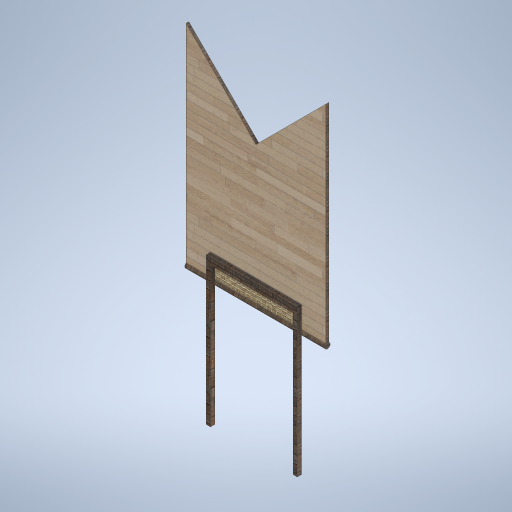
# Autodesk Inventor part: flag
Saved by Autodesk Inventor 2024.2 (Build 282272000, 272)
## iProperties
Created: 2024-05-27
Part Number: flag
Material: 一般
Document SubType Name: Modeling
Designer: user
Density: 1 g/cm^3
Appearance: 預設
Author: user
Autodesk Inventor part; units mm, degrees
ref_plane "YZ Plane" through (0, 0, 0) normal (1, 0, 0) x (0, 1, 0)
ref_plane "XZ Plane" through (0, 0, 0) normal (0, 1, 0) x (-1, 0, 0)
ref_plane "XY Plane" through (0, 0, 0) normal (0, 0, 1) x (1, 0, 0)
sketch "草圖1" plane through (0, 0, 0) normal (0, 0, 1) x (1, 0, 0)
  line L0 (-500, -500) -> (0, -1000)
  line L1 (0, -1000) -> (500, -500)
  line L2 (-500, -500) -> (-500, -2000)
  line L3 (-500, -2000) -> (500, -2000)
  line L4 (500, -2000) -> (500, -500)
  point P0 (0, 0)
  dimension "d2" = 1500
  dimension "d3" = 1000
  constraints: 10 end point, 2 perpendicular, 1 vertical
  measures "d2" distance of L0.start L2.end
  measures "d3" distance of L2.end L3.end
extrude "擠出1" add sketch "草圖1" along normal blind 20
sketch "草圖2" plane through (500, -2000, 0) normal (1, 0, 0) x (0, 0, -1)
  line L0 (0, 0) -> (-20, 0) projected
  circle A0 centre (-10, 0) radius 20
  point P0 (0, 2000)
  dimension "d6" = 40
  constraints: 1 centre point, 1 midpoint
  measures "d6" diameter of A0
extrude "擠出2" add sketch "草圖2" against normal blind 1000
sketch "草圖3" plane through (0, 0, 20) normal (0, 0, 1) x (1, 0, 0)
  line L0 (325, -1879.5485) -> (-325, -1879.5485)
  line L1 (-325, -1879.5485) -> (-325, -1829.5485)
  line L2 (-325, -1829.5485) -> (325, -1829.5485)
  line L3 (325, -1829.5485) -> (325, -1879.5485)
  line L4 (325, -1879.5485) -> (-325, -1829.5485) construction
  line L5 (-325, -1879.5485) -> (325, -1829.5485) construction
  point P0 (0, 0)
  point P1 (0, -1854.5485)
  dimension "d9" = 650
  dimension "d10" = 50
  constraints: 12 end point, 2 midpoint, 2 parallel, 1 horizontal, 1 perpendicular
  measures "d9" distance of L1.end L2.end
  measures "d10" distance of L0.end L1.end
extrude "擠出3" add sketch "草圖3" along normal blind 30
sketch "草圖4" plane through (-325, -1879.5485, 20) normal (0, -1, 0) x (1, 0, 0)
  line L0 (650, 0) -> (0, 0) projected
  line L1 (0, 30) -> (650, 30) projected
  line L2 (650, 0) -> (620, 0)
  line L3 (620, 0) -> (620, 30)
  line L4 (620, 30) -> (650, 30)
  line L5 (650, 30) -> (650, 0)
  line L6 (0, 0) -> (650, 0) projected
  line L7 (0, 30) -> (30, 30)
  line L8 (30, 30) -> (30, 0)
  line L9 (30, 0) -> (0, 0)
  line L10 (0, 0) -> (0, 30)
  point P0 (325, -20)
  dimension "d13" = 30
  dimension "d14" = 30
  constraints: 16 end point, 4 parallel, 2 horizontal, 2 perpendicular, 2 point on line
  measures "d13" distance of L3.end L4.end
  measures "d14" distance of L8.end L9.end
extrude "擠出4" add sketch "草圖4" along normal blind 1000 contours L0 L3 L1 L5
extrude "擠出5" add sketch "草圖4" along normal blind 1000 contours L0 L10 L1 L8
